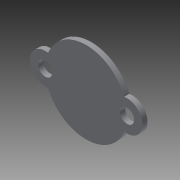
# Autodesk Inventor part: top
Saved by Autodesk Inventor 2014 (Build 180170000, 170)
## iProperties
Created: 2013-09-05
Part Number: top
Material: Generisch
Document SubType Name: Modeling
Designer: solidworks
Density: 1 g/cm^3
Appearance: Vorgabe
Author: solidworks
Autodesk Inventor part; units mm, degrees
ref_plane "YZ Plane" through (0, 0, 0) normal (1, 0, 0) x (0, 1, 0)
ref_plane "XZ Plane" through (0, 0, 0) normal (0, 1, 0) x (-1, 0, 0)
ref_plane "XY Plane" through (0, 0, 0) normal (0, 0, 1) x (1, 0, 0)
sketch "Skizze1" plane through (0, 0, 0) normal (0, 1, 0) x (-1, 0, 0)
  circle A0 centre (0, 0) radius 8
  circle A1 centre (-8, 0) radius 3
  circle A2 centre (8, 0) radius 3
  line L0 (8, 0) -> (-8, 0)
  dimension "d0" = 16
  dimension "d1" = 6
  dimension "d2" = 6
  constraints: 3 centre point, 2 end point, 2 point on circle, 1 coincident, 1 horizontal, 1 midpoint
  measures "d0" diameter of A0
  measures "d1" diameter of A1
  measures "d2" diameter of A2
extrude "Extrusion1" add sketch "Skizze1" along normal blind 1
sketch "Skizze2" plane through (0, 1, 0) normal (0, 1, 0) x (1, 0, 0)
  arc A0 (7.4375, 2.9468) -> (-7.4375, 2.9468) centre (0, 0) ccw projected
  circle A1 centre (0, 0) radius 5.875
  circle A2 centre (0, 0) radius 4.5
  dimension "d5" = 11.75
  dimension "d6" = 9
  constraints: 2 centre point, 2 coincident
  measures "d5" diameter of A1
  measures "d6" diameter of A2
extrude "Extrusion2" add sketch "Skizze2" along normal blind 0.5
sketch "Skizze3" plane through (0, 1, 0) normal (0, 1, 0) x (1, 0, 0)
  arc A0 (7.4375, -2.9468) -> (7.4375, 2.9468) centre (8, 0) ccw projected
  arc A1 (-7.4375, 2.9468) -> (-7.4375, -2.9468) centre (-8, 0) ccw projected
  circle A2 centre (-8, 0) radius 1.375
  circle A3 centre (8, 0) radius 1.375
  dimension "d9" = 2.75
  dimension "d10" = 2.75
  constraints: 2 centre point, 2 coincident
  measures "d9" diameter of A2
  measures "d10" diameter of A3
extrude "Extrusion3" cut sketch "Skizze3" against normal up to next
